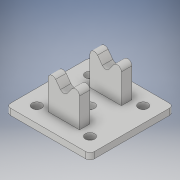
# Autodesk Inventor part: CapillaryHolder
Saved by Autodesk Inventor 2019 (Build 230136000, 136)
## iProperties
Created: 2019-07-22
Part Number: CapillaryHolder
Material: Generic
Document SubType Name: Modeling
Designer: aorfi
Density: 1 g/cm^3
Appearance: Default
Author: aorfi
Autodesk Inventor part; units mm, degrees
ref_plane "YZ Plane" through (0, 0, 0) normal (1, 0, 0) x (0, 1, 0)
ref_plane "XZ Plane" through (0, 0, 0) normal (0, 1, 0) x (-1, 0, 0)
ref_plane "XY Plane" through (0, 0, 0) normal (0, 0, 1) x (1, 0, 0)
sketch "Sketch1" plane through (0, 0, 0) normal (0, 1, 0) x (-1, 0, 0)
  line L0 (-20, 20) -> (20, 20)
  line L1 (20, 20) -> (20, -20)
  line L2 (20, -20) -> (-20, -20)
  line L3 (-20, -20) -> (-20, 20)
  line L4 (-20, 20) -> (20, -20) construction
  line L5 (20, 20) -> (-20, -20) construction
  point P0 (0, 0)
  dimension "d0" = 40
  dimension "d1" = 40
  constraints: 12 end point, 2 midpoint, 2 parallel, 1 horizontal, 1 perpendicular
  measures "d0" distance of L0.end L1.end
  measures "d1" distance of L0.start L0.end
extrude "Extrusion1" add sketch "Sketch1" along normal blind 3
sketch "Sketch2" plane through (0, 3, 0) normal (0, 1, 0) x (1, 0, 0)
  line L0 (-7.5, 12.5) -> (7.5, 12.5)
  line L1 (7.5, 12.5) -> (7.5, 7.5)
  line L2 (7.5, 7.5) -> (-7.5, 7.5)
  line L3 (-7.5, 7.5) -> (-7.5, 12.5)
  line L4 (-7.5, -7.5) -> (7.5, -7.5)
  line L5 (7.5, -7.5) -> (7.5, -12.5)
  line L6 (7.5, -12.5) -> (-7.5, -12.5)
  line L7 (-7.5, -12.5) -> (-7.5, -7.5)
  line L8 (0, 7.5) -> (0, -7.5) construction
  point P0 (-20, 20)
  point P1 (20, 20)
  point P2 (0, 0)
  point P3 (0, 0)
  dimension "d10" = 15
  dimension "d11" = 15
  dimension "d12" = 5
  constraints: 18 end point, 4 parallel, 3 midpoint, 2 collinear, 2 horizontal, 2 perpendicular, 1 coincident, 1 vertical
  measures "d10" distance between parallel lines of L4 L2
  measures "d11" distance of L0.start L0.end
  measures "d12" distance of L2.end L0.start
extrude "Extrusion2" add sketch "Sketch2" along normal blind 20
sketch "Sketch3" plane through (20, 0, -20) normal (0, 0, -1) x (-1, 0, 0)
  line L0 (40, 0) -> (0, 0) projected
  line L1 (12.5, 23) -> (27.5, 23) projected
  line L2 (12.5, 3) -> (12.5, 23) projected
  line L3 (12.5, 23) -> (20, 13)
  line L4 (20, 13) -> (27.5, 23)
  point P0 (20, 0)
  point P1 (20, 0)
  point P2 (20, 0)
  dimension "d13" = 10
  constraints: 4 end point, 2 midpoint, 1 vertical alignment
  measures "d13" distance from line of L1 L3.end
extrude "Extrusion3" cut sketch "Sketch3" against normal through all
fillet "Fillet1" radius 2 10 edges at (0, 13, 10) (0, 13, -10) (-7.5, 23, -10) (-7.5, 23, 10) (7.5, 23, 10) (7.5, 23, -10) (20, 1.5, 20) (20, 1.5, -20) (-20, 1.5, -20) (-20, 1.5, 20)
sketch "Sketch5" plane through (0, 0, 0) normal (0, -1, 0) x (1, 0, 0)
  line L0 (12.7, -12.7) -> (-12.7, -12.7) construction
  line L1 (-12.7, -12.7) -> (-12.7, 12.7) construction
  point P0 (0, 0)
  point P1 (12.7, 12.7)
  point P2 (0, -12.7)
  point P3 (-12.7, 0)
  point P4 (0, 0)
  dimension "d14" = 25.4
  dimension "d15" = 25.4
  constraints: 4 end point, 2 horizontal alignment, 2 midpoint, 2 vertical alignment, 1 coincident, 1 horizontal, 1 vertical
  measures "d14" distance of L0.start L0.end
  measures "d15" distance of L0.end L1.end
hole "Hole1" at (12.7, 0, -12.7) at (-12.7, 0, -12.7) at (12.7, 0, 12.7) at (-12.7, 0, 12.7) at (0, 0, 0) direction (0, 1, 0) diameter 4.496 end through all clearance for "Flat Head Machine Screw (82)" size "#8" standard "Ansi Unified Screw Threads"
body "Solid1"
